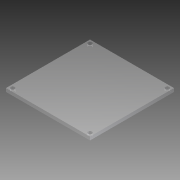
# Autodesk Inventor part: 1_0204_004
Saved by Autodesk Inventor 2012 SP1 (Build 160190100, 190)
## iProperties
Created: 2013-03-21
Part Number: 1_0204_004
Material: Default
Document SubType Name: Modeling
Designer: vogel
Density: 1 g/cm^3
Author: vogel
Autodesk Inventor part; units mm, degrees
ref_plane "YZ Plane" through (0, 0, 0) normal (1, 0, 0) x (0, 1, 0)
ref_plane "XZ Plane" through (0, 0, 0) normal (0, 1, 0) x (-1, 0, 0)
ref_plane "XY Plane" through (0, 0, 0) normal (0, 0, 1) x (1, 0, 0)
sketch "Skizze1" plane through (0, 0, 0) normal (0, 0, 1) x (1, 0, 0)
  line L0 (0, 0) -> (50, 0)
  line L1 (50, 0) -> (50, 50)
  line L2 (50, 50) -> (0, 50)
  line L3 (0, 50) -> (0, 0)
  dimension "d0" = 50
  dimension "d1" = 50
  constraints: 8 end point, 2 parallel, 1 horizontal, 1 perpendicular
  measures "d0" distance of L2.end L0.start
  measures "d1" distance of L0.start L0.end
extrude "Extrusion1" add sketch "Skizze1" along normal blind 2
sketch "Skizze3" plane through (0, 0, 2) normal (0, 0, 1) x (1, 0, 0)
  line L0 (0, 0) -> (0, 50) projected
  line L1 (50, 0) -> (0, 0) projected
  line L2 (50, 50) -> (50, 0) projected
  line L3 (0, 50) -> (50, 50) projected
  line L4 (2, 48) -> (2, 2)
  line L5 (2, 2) -> (48, 2)
  line L6 (48, 2) -> (48, 48)
  line L7 (48, 48) -> (2, 48)
  dimension "d15" = 2
  constraints: 8 end point, 4 coincident, 3 other
  measures "d15" distance between parallel lines of L0 L4
hole "Bohrung2" at (2, 48, 2) at (48, 48, 2) at (48, 2, 2) at (2, 2, 2) direction (0, 0, -1) diameter 2.4 end through all
